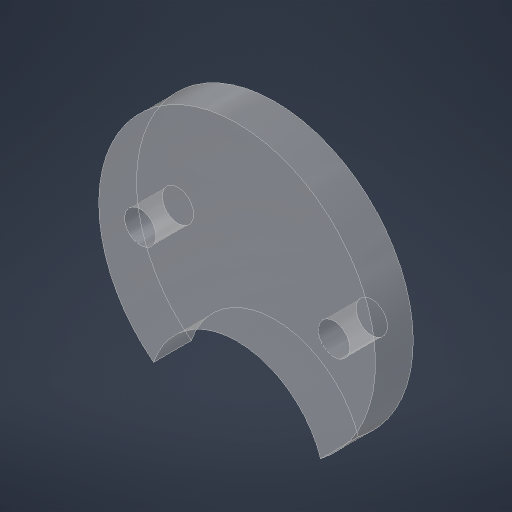
# Autodesk Inventor part: Caster Spacer 3mm
Saved by Autodesk Inventor 2026.1 (Build 301233020, 233B)
## iProperties
Created: 2020-09-02
Part Number: Caster Spacer 3mm
Material: PMMA Plastic
Document SubType Name: Modeling
Designer: Mike Angus
Density: 1.188 g/cm^3
Appearance: Polycarbonate - Clear
cs_holeSpacing: 15,400 mm
cs_holeDiam: 2,500 mm
cs_diam: 22,000 mm
Author: Mike Angus
Autodesk Inventor part; units mm, degrees
ref_plane "YZ Plane" through (0, 0, 0) normal (1, 0, 0) x (0, 1, 0)
ref_plane "XZ Plane" through (0, 0, 0) normal (0, 1, 0) x (-1, 0, 0)
ref_plane "XY Plane" through (0, 0, 0) normal (0, 0, 1) x (1, 0, 0)
sketch "Sketch1" plane through (0, 0, 0) normal (0, 0, 1) x (1, 0, 0)
  circle A0 centre (0, 0) radius 11
  line L0 (-7.7, 0) -> (7.7, 0) construction
  circle A1 centre (-7.7, 0) radius 1.25
  circle A2 centre (7.7, 0) radius 1.25
  dimension "d0" = 22
  dimension "d1" = 15.4
  dimension "d2" = 2.5
  dimension "d3" = 2.5
  constraints: 4 coincident, 3 centre point, 2 end point, 1 horizontal, 1 midpoint
  measures "d0" diameter of A0
  measures "d1" distance of L0.start L0.end
  measures "d2" diameter of A1
  measures "d3" diameter of A2
extrude "Extrusion1" add sketch "Sketch1" along normal blind 3
sketch "Sketch2" plane through (0, 0, 3) normal (0, 0, 1) x (1, 0, 0)
  circle A0 centre (0, 0) radius 11 projected
  arc A1 (6.6742, -8.8894) -> (0, -4) centre (0, -11) ccw
  arc A2 (0, -4) -> (-6.6426, -8.7919) centre (0, -11) ccw
  point P0 (-6.6362, -8.7727)
  point P1 (6.6362, -8.7727)
  constraints: 4 point on circle, 2 centre point, 1 coincident, 2 other
extrude "Extrusion2" cut sketch "Sketch2" against normal blind 10 contours A2 A1 A0 picked at (-1.3613, -8.6538)
equation "\"d0\" = cs_diam"
equation "\"d1\" = cs_holeSpacing"
equation "\"d2\" = cs_holeDiam"
equation "\"d3\" = cs_holeDiam"
equation "\"d4\" = cs_depth"
equation "\"cs_diam\" = 22"
equation "\"cs_holeSpacing\" = 15.4"
equation "\"cs_holeDiam\" = 2.5"
equation "\"cs_depth\" = 3"
body "Solid1"
